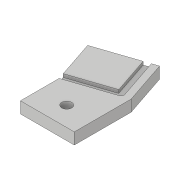
# Autodesk Inventor part: Lidar Sensor Case Piece 2
Saved by Autodesk Inventor 2018.3 (Build 223284000, 284)
## iProperties
Created: 2019-02-26
Part Number: Lidar Sensor Case Piece 2
Material: Generic
Document SubType Name: Modeling
Designer: aye06091
Mass: 6.65378 g
Surface Area: 34.8257 cm^2
Volume: 6.65378 cm^3
Density: 1 g/cm^3
Appearance: Default
Author: aye06091
Autodesk Inventor part; units mm, degrees
ref_plane "YZ Plane" through (0, 0, 0) normal (1, 0, 0) x (0, 1, 0)
ref_plane "XZ Plane" through (0, 0, 0) normal (0, 1, 0) x (-1, 0, 0)
ref_plane "XY Plane" through (0, 0, 0) normal (0, 0, 1) x (1, 0, 0)
sketch "Sketch1" plane through (0, 0, 0) normal (0, 1, 0) x (-1, 0, 0)
  line L0 (-8.0312, -19.6194) -> (-8.0312, -0.5694)
  line L1 (-8.0312, -0.5694) -> (-34.5277, -0.5694)
  line L2 (-34.5277, -0.5694) -> (-34.5277, -28.5056)
  line L3 (18.6455, 5.0782) -> (18.6456, 5.0782)
  line L4 (-1.974, -37.6808) -> (-8.0312, -19.6194)
  line L5 (-34.5277, -28.5056) -> (-27.4611, -49.5771)
  line L6 (-1.974, -37.6808) -> (-0.9645, -40.691)
  line L7 (-27.4611, -49.5771) -> (-0.9645, -40.691)
  circle A0 centre (-21.2794, -10.0945) radius 2.4447
  line L8 (-8.0312, -0.5694) -> (-8.0312, -19.6194)
  line L9 (-8.0312, -19.6194) -> (-0.9645, -40.691)
  line L10 (-0.9645, -40.691) -> (-27.4611, -49.5771)
  line L11 (-27.4611, -49.5771) -> (-34.5277, -28.5056)
  line L12 (-34.5277, -28.5056) -> (-34.5277, -0.5694)
  line L13 (-34.5277, -0.5694) -> (-8.0312, -0.5694)
  point P0 (0, 0)
  dimension "d0" = 19.05
  dimension "d1" = 22.225
  dimension "d2" = 27.9469
  dimension "d3" = 26.4965
  dimension "d4" = 4.8895
  constraints: 28 end point, 3 perpendicular, 2 parallel, 1 centre point, 1 collinear, 1 vertical
  measures "d0" distance of L0.start L0.end
  measures "d1" distance of L4.end L6.end
  measures "d2" distance of L5.end L7.end
  measures "d3" distance of L0.end L1.end
  measures "d4" diameter of A0
extrude "Extrusion1" add sketch "Sketch1" along normal blind 5.6134
sketch "Sketch2" plane through (0, 5.6134, 0) normal (0, 1, 0) x (1, 0, 0)
  line L0 (31.5176, 27.4961) -> (8.0312, 19.6194)
  line L1 (8.0312, 19.6194) -> (7.0136, 22.6537)
  line L2 (7.0136, 22.6537) -> (27.4657, 29.5128)
  line L3 (31.5176, 27.4961) -> (29.9884, 26.9832)
  line L4 (27.4657, 29.5128) -> (21.4165, 47.5499)
  line L5 (21.4165, 47.5499) -> (24.4508, 48.5676)
  line L6 (24.4508, 48.5676) -> (31.5176, 27.4961)
  line L7 (27.4611, 49.5771) -> (0.9645, 40.691) projected
  point P0 (0, 0)
  point P1 (0, 0)
  dimension "d10" = 3.175
  dimension "d11" = 3.2004
  dimension "d12" = 3.2004
  dimension "d15" = 0
  constraints: 14 end point, 3 parallel, 2 perpendicular, 1 point on line
  measures "d10" distance from line of L7.start L6
  measures "d11" distance between parallel lines of L2 L0
  measures "d12" distance between parallel lines of L6 L4
  measures "d15" distance from line of L7 L4.end
extrude "Extrusion2" cut sketch "Sketch2" against normal blind 1.5875
fillet "Fillet1" radius 1.5875 1 edges at (31.5176, 4.8197, -27.4961)
body "Solid1"
